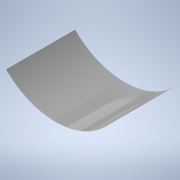
# Autodesk Inventor part: Chapa_Inox
Saved by Autodesk Inventor 2022 (Build 260153000, 153)
## iProperties
Created: 2016-02-19
Part Number: Chapa_Inox
Material: Aço AISI 1020 107 HR
Document SubType Name: Modeling
Designer: al131100X
Density: 7.87 g/cm^3
Appearance: Aço
Mass: 9955.13 g
Surface Area: 50630.6 cm^2
Volume: 1264.95 cm^3
Author: al131100X
Autodesk Inventor part; units mm, degrees
ref_plane "YZ Plane" through (0, 0, 0) normal (1, 0, 0) x (0, 1, 0)
ref_plane "XZ Plane" through (0, 0, 0) normal (0, 1, 0) x (-1, 0, 0)
ref_plane "XY Plane" through (0, 0, 0) normal (0, 0, 1) x (1, 0, 0)
sketch "Sketch1" plane through (0, 0, 0) normal (0, 1, 0) x (-1, 0, 0)
  arc A0 (2077.6508, 261.5825) -> (3884.0249, 266.2038) centre (2978.5428, 1160.9837) ccw
  arc A1 (2078.0046, 261.9358) -> (3878.0043, 260.8586) centre (2978.5428, 1160.9837) ccw
  line L0 (2077.6508, 261.5825) -> (2078.0046, 261.9358)
  line L1 (3884.0249, 266.2038) -> (3883.6714, 266.5574)
  arc A2 (2078.0046, 261.9358) -> (3883.6714, 266.5574) centre (2978.5428, 1160.9837) ccw
  point P0 (0, 0)
  dimension "d9" = 0.5
  dimension "d16" = 1800
  dimension "d22" = 1273
  constraints: 6 point on circle, 4 end point, 3 centre point, 1 coincident, 1 concentric, 1 other
  measures "d9" radial gap between concentric circles of A0 A1
  measures "d16" distance of A1.end L0.end
  measures "d22" radius of A0
extrude "Extrusion1" add sketch "Sketch1" along normal blind 1260
body "Solid1"
